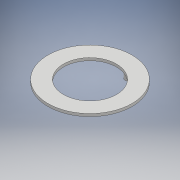
# Autodesk Inventor part: Medio Circulo
Saved by Autodesk Inventor 2018 (Build 220112000, 112)
## iProperties
Created: 2018-04-04
Part Number: Medio Circulo
Material: Générique
Document SubType Name: Modeling
Designer: Guadalix
Density: 1 g/cm^3
Appearance: Par défaut
Author: Guadalix
Autodesk Inventor part; units mm, degrees
ref_plane "YZ Plane" through (0, 0, 0) normal (1, 0, 0) x (0, 1, 0)
ref_plane "XZ Plane" through (0, 0, 0) normal (0, 1, 0) x (-1, 0, 0)
ref_plane "XY Plane" through (0, 0, 0) normal (0, 0, 1) x (1, 0, 0)
sketch "Esquisse1" plane through (0, 0, 0) normal (0, 0, 1) x (1, 0, 0)
  circle A0 centre (0, 0) radius 47.5
  circle A1 centre (0, 0) radius 30
  point P0 (0, 45)
  point P1 (0, 47.5)
  dimension "d0" = 95
  dimension "d1" = 60
  dimension "d2" = 2.5
  constraints: 2 coincident, 1 centre point, 1 vertical alignment, 2 other
  measures "d1" diameter of A1
  measures "d2" distance of point (0, 45) point (0, 47.5)
sketch "Esquisse2" plane through (0, 0, 0) normal (0, 0, 1) x (1, 0, 0)
  circle A0 centre (0, 43.6003) radius 3.0751
  point P0 (0, 0)
  constraints: 1 centre point
extrude "Extrusion1" add sketch "Esquisse1" along normal blind 3
extrude "Extrusion2" cut sketch "Esquisse2" along normal blind 2
sketch "Esquisse3" plane through (0, 43.6003, 2) normal (0, 0, -1) x (-1, 0, 0)
  circle A0 centre (0, 0) radius 3.0751 projected
  line L0 (-1, 2.908) -> (-1, 1.908)
  line L1 (-1, 1.908) -> (1, 1.908)
  line L2 (1, 1.908) -> (1, 2.908)
  arc A1 (1, 2.908) -> (-1, 2.908) centre (0, 0) ccw
  line L3 (-1, -2.908) -> (-1, -1.908)
  line L4 (-1, -1.908) -> (1, -1.908)
  line L5 (1, -1.908) -> (1, -2.908)
  arc A2 (-1, -2.908) -> (1, -2.908) centre (0, 0) ccw
  circle A3 centre (0, 0) radius 3.9
  point P0 (0, -43.6003)
  dimension "d7" = 2
  dimension "d8" = 1
  dimension "d9" = 1
  dimension "d10" = 2
  dimension "d11" = 1
  dimension "d12" = 1
  dimension "d13" = 7.8
  constraints: 12 end point, 8 point on circle, 4 perpendicular, 3 centre point, 2 concentric, 2 vertical, 1 coincident
  measures "d7" distance between parallel lines of L2 L0
  measures "d8" distance from line of A0.centre L0
  measures "d9" distance from line of L2.end L1
  measures "d10" distance between parallel lines of L5 L3
  measures "d11" distance from line of A0.centre L5
  measures "d12" distance from line of L3.start L4
  measures "d13" diameter of A3
extrude "Extrusion3" add sketch "Esquisse3" along normal blind 20 contours L2 L1 L0 A0 | A0 L3 L4 L5 | A3
